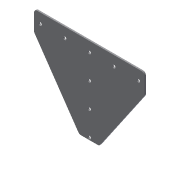
# Autodesk Inventor part: super4
Saved by Autodesk Inventor 2015 SP1 (Build 190203100, 203)
## iProperties
Created: 2015-01-18
Part Number: super4
Material: Generic
Document SubType Name: Sheet Metal
Designer: Owner
Density: 1 g/cm^3
Sheet Metal Rule: Default
Appearance: Default
Author: Owner
Autodesk Inventor part; units mm, degrees
ref_plane "YZ Plane" through (0, 0, 0) normal (1, 0, 0) x (0, 1, 0)
ref_plane "XZ Plane" through (0, 0, 0) normal (0, 1, 0) x (-1, 0, 0)
ref_plane "XY Plane" through (0, 0, 0) normal (0, 0, 1) x (1, 0, 0)
sketch "Sketch1" plane through (0, 0, 0) normal (0, 0, 1) x (1, 0, 0)
  line L0 (0, 0) -> (228.6, 0)
  line L1 (0, 0) -> (0, -41.402)
  line L2 (228.6, 0) -> (228.6, -41.402)
  line L3 (93.599, -177.8) -> (135.001, -177.8)
  line L4 (0, -41.402) -> (93.599, -177.8)
  line L5 (228.6, -41.402) -> (135.001, -177.8)
  circle A0 centre (215.9, -20.701) radius 3.3655
  circle A1 centre (165.1, -20.701) radius 3.3655
  circle A2 centre (114.3, -20.701) radius 3.3655
  circle A3 centre (63.5, -20.701) radius 3.3655
  circle A4 centre (12.7, -20.701) radius 3.3655
  line L6 (114.3, 0) -> (114.3, -20.701)
  circle A5 centre (114.3, -71.501) radius 3.3655
  circle A6 centre (114.3, -122.301) radius 3.3655
  circle A7 centre (114.3, -173.101) radius 3.3655
  dimension "d0" = 228.6
  dimension "d6" = 41.402
  dimension "d7" = 41.402
  dimension "d8" = 41.402
  dimension "d9" = 177.8
  dimension "d11" = 93.599
  dimension "d13" = 6.731
  dimension "d14" = 12.7
  dimension "d15" = 20.701
  dimension "d18" = 50.8
  dimension "d25" = 50.8
  measures "d0" distance of L0.start L0.end
  measures "d6" distance of L0.end L2.end
  measures "d7" distance of L0.start L1.end
  measures "d8" distance of L3.start L3.end
  measures "d9" distance between parallel lines of L3 L0
  measures "d11" horizontal distance of L3.start point (0, 0)
  measures "d13" diameter of A0
  measures "d14" distance from line of A0.centre L2
  measures "d15" distance from line of A0.centre L0
  measures "d18" distance of A0.centre A1.centre
  measures "d25" distance of L6.end A5.centre
extrude "Plate1" add sketch "Sketch1" along normal blind 3.048
fillet "Corner Round1" radius 6.35 6 edges at (0, 0, 1.524) (0, -41.402, 1.524) (228.6, 0, 1.524) (228.6, -41.402, 1.524) (135.001, -177.8, 1.524) (93.599, -177.8, 1.524)
equation "\"d15\" = 0.5 * d6"
equation "\"BendRadius\" = Thickness"
equation "\"BendReliefWidth\" = Thickness"
equation "\"BendReliefDepth\" = 0.5 * Thickness"
equation "\"CornerReliefSize\" = 4 * Thickness"
equation "\"MinimumRemnant\" = 2 * Thickness"
equation "\"TransitionRadius\" = BendRadius"
equation "\"JacobiRadiusSize\" = BendRadius"
equation "\"GapSize\" = Thickness"
equation "\"d30\" = BendRadius"
equation "\"Thickness\" = 3.048"
body "Solid1"
